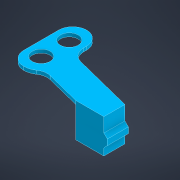
# Autodesk Inventor part: Ultrasonic Gantry
Saved by Autodesk Inventor 2022 (Build 260153000, 153)
## iProperties
Created: 2021-05-30
Part Number: Ultrasonic Gantry
Material: Generic
Document SubType Name: Modeling
Designer: sidsa
Density: 1 g/cm^3
Appearance: Sky Blue Medium
Author: sidsa
## iProperties of the stored document Ultrasonic Gantry_3DPrint.ipt
Created: 2021-05-30
Part Number: Ultrasonic Gantry_3DPrint
Material: Generic
Document SubType Name: Modeling
Designer: sidsa
Density: 1 g/cm^3
Appearance: Default
Author: sidsa
Autodesk Inventor part; units mm, degrees
ref_plane "YZ Plane" through (0, 0, 0) normal (1, 0, 0) x (0, 1, 0)
ref_plane "XZ Plane" through (0, 0, 0) normal (0, 1, 0) x (-1, 0, 0)
ref_plane "XY Plane" through (0, 0, 0) normal (0, 0, 1) x (1, 0, 0)
sketch "Sketch1" plane through (0, 0, 0) normal (0, 0, 1) x (1, 0, 0)
  line L0 (0, 0) -> (3.175, 0)
  line L1 (3.175, 0) -> (3.175, 18.3388)
  line L2 (3.175, 18.3388) -> (0, 18.3388)
  line L3 (0, 18.3388) -> (0, 0)
  dimension "d0" = 3.175
  dimension "d1" = 18.3388
  constraints: 8 end point, 2 parallel, 1 horizontal, 1 perpendicular
  measures "d0" distance of L2.end L1.end
  measures "d1" distance of L0.end L1.end
extrude "Extrusion1" add sketch "Sketch1" along normal blind 16.002
sketch "Sketch2" plane through (0, 0, 16.002) normal (0, 0, 1) x (1, 0, 0)
  line L0 (3.175, 18.3388) -> (-22.225, 18.3388)
  line L1 (-22.225, 18.3388) -> (-22.225, 0)
  line L2 (-22.225, 0) -> (3.175, 0)
  line L3 (3.175, 0) -> (3.175, 18.3388)
  line L4 (3.175, 0) -> (3.175, 18.3388) construction
  line L5 (3.175, 18.3388) -> (0, 18.3388) construction
  line L6 (0, 18.3388) -> (0, 0) construction
  line L7 (0, 0) -> (3.175, 0) construction
  line L8 (3.175, 0) -> (3.175, 18.3388) projected
  line L9 (3.175, 18.3388) -> (0, 18.3388) projected
  dimension "d4" = 25.4
  constraints: 8 end point, 2 collinear, 2 parallel, 1 horizontal, 1 perpendicular
  measures "d4" distance of L1.end L2.end
extrude "Extrusion2" add sketch "Sketch2" along normal blind 3.175
sketch "Sketch3" plane through (0, 18.3388, 0) normal (0, 1, 0) x (1, 0, 0)
  line L0 (3.175, 0) -> (3.175, -19.177) projected
  line L1 (3.175, -19.177) -> (-22.225, -19.177)
  line L2 (-22.225, -19.177) -> (-22.225, 0)
  line L3 (-22.225, 0) -> (3.175, 0)
  line L4 (3.175, 0) -> (3.175, -19.177)
  line L5 (-22.225, -16.002) -> (-22.225, -19.177) projected
  point P0 (0, 0)
  constraints: 8 end point, 2 parallel, 1 collinear, 1 horizontal, 1 perpendicular
extrude "Extrusion3" add sketch "Sketch3" along normal blind 9.525
sketch "Sketch4" plane through (0, 27.8638, 0) normal (0, 1, 0) x (1, 0, 0)
  line L0 (3.175, 0) -> (3.175, -19.177) projected
  line L1 (3.175, -19.177) -> (-22.225, -19.177)
  line L2 (-22.225, -19.177) -> (-22.225, 12.7) construction
  line L3 (-22.225, 12.7) -> (3.175, 12.7) construction
  line L4 (3.175, 12.7) -> (3.175, -19.177) construction
  line L5 (-22.225, 0) -> (-22.225, -19.177) construction
  line L6 (3.175, 0) -> (-22.225, 0) construction
  line L7 (3.175, 12.7) -> (-73.025, 12.7)
  line L8 (-60.325, 34.925) -> (-60.325, -9.525)
  line L9 (-60.325, -9.525) -> (-85.725, -9.525)
  line L10 (-85.725, -9.525) -> (-85.725, 34.925)
  line L11 (-85.725, 34.925) -> (-60.325, 34.925)
  line L12 (-60.325, 34.925) -> (-85.725, -9.525) construction
  line L13 (-60.325, -9.525) -> (-85.725, 34.925) construction
  line L14 (-73.025, 34.925) -> (-73.025, -9.525) construction
  circle A0 centre (-73.025, -0.1016) radius 8.128
  circle A1 centre (-73.025, 25.5016) radius 8.128
  line L15 (-22.225, -19.177) -> (3.175, -19.177) projected
  line L16 (-22.225, -19.177) -> (-60.325, -9.525)
  line L17 (0, 0) -> (3.175, 0) projected
  line L18 (3.175, 0) -> (-60.325, 16.0867)
  circle A2 centre (-73.025, -0.1016) radius 15.8142
  circle A3 centre (-73.025, 25.5016) radius 15.8142
  point P0 (-60.325, 34.925)
  point P1 (-85.725, -9.525)
  dimension "d9" = 12.7
  dimension "d10" = 76.2
  dimension "d11" = 44.45
  dimension "d12" = 25.4
  dimension "d13" = 16.256
  dimension "d14" = 12.8016
  constraints: 28 end point, 5 parallel, 4 midpoint, 2 centre point, 2 coincident, 2 horizontal, 2 perpendicular, 2 point on line, 1 collinear, 1 symmetric about line, 1 vertical, 7 other
  measures "d9" distance between parallel lines of L6 L3
  measures "d10" distance of L3.end L7.end
  measures "d11" distance of L8.start L8.end
  measures "d12" distance of L8.end L9.end
  measures "d13" diameter of A0
  measures "d14" distance of L7.end A0.centre
extrude "Extrusion4" add sketch "Sketch4" along normal blind 3.175 contours L0 L1 L16 A2 L8 L7 L18 | L7 L8 L18 | L8 A2 L7 | L7 A3 L8 | A3 A2 L10 L11 L8 | L9 L10 A2 A3 L8 | A2 L9 | L8 A2 | A3 A2 | L11 A3 | A2 L10 A3
fillet "Fillet1" radius 12.7 5 edges at (-60.325, 29.4513, -16.0867) (-60.325, 29.4513, -34.925) (-85.725, 29.4513, -34.925) (-60.325, 29.4513, 9.525) (-85.725, 29.4513, 9.525)
sketch "Sketch5" plane through (3.175, 0, 19.177) normal (1, 0, 0) x (0, 0, -1)
  line L0 (0, 31.0388) -> (19.177, 31.0388) construction
  line L1 (0, 0) -> (0, 31.0388) construction
  line L2 (19.177, 0) -> (19.177, 27.8638) construction
  line L3 (19.177, 0) -> (0, 0) construction
  line L4 (0, 18.1388) -> (19.177, 18.1388)
  line L5 (19.177, 18.1388) -> (19.177, 6.5388)
  line L6 (19.177, 6.5388) -> (0, 6.5388)
  line L7 (0, 6.5388) -> (0, 18.1388)
  line L8 (20.977, 18.1388) -> (19.377, 18.1388)
  line L9 (19.377, 6.5388) -> (20.977, 6.5388)
  line L10 (0, 18.1388) -> (19.177, 18.1388)
  line L11 (19.177, 18.1388) -> (19.177, 6.5388)
  line L12 (19.177, 6.5388) -> (0, 6.5388)
  line L13 (0, 6.5388) -> (0, 18.1388)
  point P0 (19.177, 0)
  constraints: 28 end point, 4 parallel, 2 collinear, 2 horizontal, 2 perpendicular, 2 point on line
extrude "Extrusion5" add sketch "Sketch5" along normal blind 3.175
chamfer "Chamfer1" distance 3.175 angle 45 2 edges at (6.35, 18.1388, 9.5885) (6.35, 6.5388, 9.5885)
sketch "Sketch6" plane through (0, 0, 0) normal (0, 0, -1) x (-1, 0, 0)
  arc A0 (-1.9233, 11.4351) -> (-1.828, 11.4908) centre (-2.3876, 12.3388) ccw
  circle A1 centre (-2.3876, 12.3388) radius 1.016
  line L0 (-6.35, 9.7138) -> (-6.35, 14.9638) projected
  line L1 (0, 18.3388) -> (0, 0) construction
  line L2 (22.225, 0) -> (0, 0) construction
  line L3 (22.225, 18.3388) -> (22.225, 0) construction
  line L4 (0, 18.3388) -> (22.225, 18.3388) construction
  line L5 (-3.175, 6.5388) -> (-6.35, 9.7138) construction
  line L6 (-3.175, 0) -> (-3.175, 6.5388) construction
  line L7 (0, 0) -> (-3.175, 0) construction
  line L8 (0, 18.3388) -> (0, 0) construction
  line L9 (0, 18.3388) -> (22.225, 18.3388) construction
  line L10 (22.225, 18.3388) -> (22.225, 27.8638) construction
  line L11 (-3.175, 27.8638) -> (22.225, 27.8638) construction
  line L12 (-3.175, 18.1388) -> (-3.175, 27.8638) construction
  line L13 (-6.35, 14.9638) -> (-3.175, 18.1388) construction
  line L14 (-6.35, 9.7138) -> (-6.35, 14.9638) construction
  line L15 (-6.35, 12.3388) -> (3.3146, 12.3388)
  point P0 (-1.9233, 11.4351)
  point P1 (-1.828, 11.4908)
  dimension "d23" = 3.9624
  dimension "d24" = 2.032
  dimension "d25" = 0
  constraints: 2 centre point, 2 end point, 2 point on circle, 1 coincident, 1 concentric, 1 horizontal, 1 midpoint
  measures "d23" distance from line of L0 A1.centre
  measures "d24" diameter of A1
  measures "d25" distance from line of L15 A0.centre
extrude "Extrusion6" cut sketch "Sketch6" against normal blind 12.7
sketch "Sketch7" plane through (0, 27.8638, 0) normal (0, -1, 0) x (1, 0, 0)
  arc A0 (-73.025, 15.9158) -> (-85.725, 3.2158) centre (-73.025, 3.2158) ccw projected
  line L0 (-85.725, -28.6158) -> (-85.725, 3.2158) projected
  arc A1 (-85.725, -28.6158) -> (-60.325, -28.6158) centre (-73.025, -28.6158) ccw projected
  line L1 (-60.325, -25.9705) -> (-60.325, -28.6158) projected
  arc A2 (-50.7438, -13.6594) -> (-60.325, -25.9705) centre (-47.625, -25.9705) ccw projected
  line L2 (3.175, 0) -> (-50.7438, -13.6594) projected
  line L3 (3.175, 0) -> (-22.225, 0) projected
  line L4 (-22.225, 0) -> (-22.225, 19.177) projected
  line L5 (-53.649, 11.2163) -> (-22.225, 19.177) projected
  arc A3 (-64.0086, 13.0937) -> (-53.649, 11.2163) centre (-56.7678, 23.5273) ccw projected
  arc A4 (-64.0086, 13.0937) -> (-73.025, 15.9158) centre (-73.025, 0.1016) ccw projected
  circle A5 centre (-73.025, -25.5016) radius 8.128 projected
  circle A6 centre (-73.025, 0.1016) radius 8.128 projected
  arc A7 (-50.7438, -13.6594) -> (-60.325, -25.9705) centre (-47.625, -25.9705) ccw projected
  line L6 (-50.7438, -13.6594) -> (-69.1935, -18.3333)
  circle A8 centre (-73.025, -25.5016) radius 8.128 projected
  circle A9 centre (-73.025, 0.1016) radius 8.128 projected
  line L7 (-71.029, -7.7775) -> (-22.225, 4.5862)
  line L8 (-73.025, -8.0264) -> (-85.725, -8.0264)
  line L9 (-73.025, -17.3736) -> (-85.725, -17.3736)
  line L10 (-85.725, -28.6158) -> (-85.725, 3.2158) projected
  point P0 (0, 0)
  point P1 (-71.029, -7.7775)
  constraints: 8 end point, 4 point on circle, 3 point on line, 2 parallel, 2 tangent, 1 collinear, 1 perpendicular
extrude "Extrusion7" add sketch "Sketch7" along normal blind 3.175 contours L8 A6 L7 L4 L3 L2 L6 A5 L9 L0
chamfer "Chamfer2" distance 3.175 angle 45 6 edges at (-79.375, 24.6888, -8.0264) (-72.0193, 24.6888, -7.9639) (-46.627, 24.6888, -1.5957) (-79.375, 24.6888, -17.3736) (-71.0501, 24.6888, -17.6172) (-33.0092, 24.6888, -9.1667)
body "Solid1"
